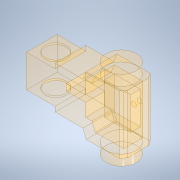
# Autodesk Inventor part: body_2
Saved by Autodesk Inventor 2020.2 (Build 242310000, 310)
## iProperties
Created: 2021-03-27
Part Number: body_2
Material: Generic
Document SubType Name: Modeling
Designer: DELL
Density: 1 g/cm^3
Appearance: Clear - Blue(1)
Author: DELL
Autodesk Inventor part; units mm, degrees
ref_plane "YZ Plane" through (0, 0, 0) normal (1, 0, 0) x (0, 1, 0)
ref_plane "XZ Plane" through (0, 0, 0) normal (0, 1, 0) x (-1, 0, 0)
sketch "Sketch1" plane through (0, 0, 0) normal (0, 0, 1) x (1, 0, 0)
  line L0 (-100, 0) -> (100, 0) construction
  line L1 (-100, 65) -> (-100, -65)
  circle A0 centre (-52.5, 57.5) radius 2.25
  line L2 (100, -70) -> (100, 70) construction
  line L3 (-92, 0) -> (-92, 57.5) construction
  line L4 (-92, 0) -> (-92, -57.5) construction
  circle A1 centre (-92.5, 57.5) radius 2.25
  circle A2 centre (-92.5, 57.5) radius 1.25
  circle A3 centre (-52.5, 57.5) radius 1.25
  line L5 (-100, 65) -> (-22.5777, 65)
  line L6 (-22.5777, 65) -> (-12.5777, 90)
  line L7 (-12.5777, 90) -> (100, 90)
  line L8 (100, 90) -> (100, 0)
  line L9 (100, -90) -> (100, 0)
  line L10 (-12.5777, -90) -> (100, -90)
  line L11 (-22.5777, -65) -> (-12.5777, -90)
  line L12 (-100, -65) -> (-22.5777, -65)
  line L13 (85, 75) -> (-2.4223, 75)
  line L14 (-2.4223, 75) -> (-12.4223, 50)
  line L15 (-12.4223, 50) -> (-92, 50)
  line L16 (-92, -50) -> (-12.4223, -50)
  line L17 (-12.4223, -50) -> (-2.4223, -75)
  line L18 (-2.4223, -75) -> (85, -75)
  line L19 (92.5, 82.5) -> (-7.5, 82.5) construction
  line L20 (-7.5, 82.5) -> (-17.5, 57.5) construction
  line L21 (-17.5, 57.5) -> (-92.5, 57.5) construction
  line L22 (-92.5, 57.5) -> (-92.5, -57.5) construction
  line L23 (-92.5, -57.5) -> (-17.5, -57.5) construction
  line L24 (-17.5, -57.5) -> (-7.5, -82.5) construction
  line L25 (-7.5, -82.5) -> (92.5, -82.5) construction
  line L26 (92.5, -82.5) -> (92.5, 0) construction
  line L27 (92.5, 0) -> (92.5, 82.5) construction
  line L28 (85, 75) -> (85, -75)
  line L29 (-100, 65) -> (-108, 65)
  line L30 (-108, 65) -> (-108, -65)
  line L31 (-108, -65) -> (-100, -65)
  line L32 (-100, -65) -> (-100, 65)
  line L33 (100, 0) -> (-108, 0)
  circle A4 centre (20, 82.5) radius 1.25
  circle A5 centre (20, 82.5) radius 2.25
  circle A6 centre (80, 82.5) radius 1.25
  circle A7 centre (80, 82.5) radius 2.25
  line L34 (50, 90) -> (50, 75) construction
  circle A8 centre (-12.5, 70) radius 1.25
  circle A9 centre (-12.5, 70) radius 2.25
  line L35 (-92, 50) -> (-92, -50)
  circle A10 centre (-96, 0) radius 2.25
  circle A11 centre (-96, 0) radius 1.25
  circle A12 centre (-104, 30) radius 2.25
  circle A13 centre (-104, 30) radius 1.25
  circle A14 centre (-104, -30) radius 2.25
  circle A15 centre (-104, -30) radius 1.25
  line L36 (-104, 65) -> (-104, -65) construction
  line L37 (-32, 50) -> (-32, 10)
  line L38 (-32, 10) -> (-92, 10)
  line L39 (77, 0) -> (77, -50)
  line L40 (77, -50) -> (-3, -50)
  line L41 (-3, -50) -> (-3, 0)
  line L42 (77, -40) -> (67, -40)
  line L43 (67, -40) -> (67, -50)
  line L44 (27, -50) -> (27, -40)
  line L45 (27, -40) -> (17, -40)
  line L46 (17, -40) -> (17, -50)
  circle A16 centre (57, 0) radius 7.5
  point P0 (0, 0)
  point P1 (0, 0)
  point P2 (77, 0)
  point P3 (-3, 0)
  dimension "d0" = 130
  dimension "d1" = 8
  dimension "d2" = 200
  dimension "d15" = 15
  dimension "d17" = 7.5
  dimension "d18" = 4.5
  dimension "d19" = 2.5
  dimension "d20" = 40
  dimension "d21" = 180
  dimension "d22" = 15
  dimension "d24" = 8
  dimension "d28" = 20
  dimension "d29" = 50
  dimension "d30" = 40
  dimension "d40" = 30
  dimension "d41" = 4
  dimension "d110" = 40
  dimension "d111" = 60
  dimension "d114" = 10
  dimension "d115" = 8
  dimension "d132" = 50
  dimension "d133" = 80
  dimension "d135" = 15
  dimension "d138" = 20
  dimension "d139" = 29
  dimension "d140" = 40
  dimension "d141" = 10
  constraints: 94 end point, 21 point on line, 17 centre point, 14 equal radius, 10 coincident, 8 perpendicular, 7 midpoint, 6 parallel, 6 symmetric about line, 4 vertical, 3 collinear, 3 equal length, 3 horizontal, 16 other
  measures "d0" distance of L29.start L12.start
  measures "d1" distance between parallel lines of L1 L3
  measures "d2" distance between parallel lines of L1 L2
  measures "d15" distance between parallel lines of L7 L13
  measures "d17" distance between parallel lines of L7 L19
  measures "d18" diameter of A1
  measures "d19" diameter of A2
  measures "d20" distance of A1.centre A3.centre
  measures "d21" distance between parallel lines of L10 L7
  measures "d22" distance between parallel lines of L9 L28
  measures "d24" distance between parallel lines of L1 L30
  measures "d28" distance from line of L8 A6.centre
  measures "d29" distance between parallel lines of L8 L34
  measures "d30" horizontal distance of A3.centre A8.centre
  measures "d40" distance from line of L33 A12.centre
  measures "d41" distance from line of L1 A10.centre
  measures "d110" distance of L37.start L37.end
  measures "d111" distance of L37.end L38.end
  measures "d114" distance of L42.end L43.end
  measures "d115" distance between parallel lines of L39 L28
  measures "d132" distance between parallel lines of L40 L0
  measures "d133" distance between parallel lines of L39 L41
  measures "d135" diameter of A16
  measures "d138" distance from line of L39 A16.centre
  measures "d139" distance between parallel lines of L37 L41
  measures "d140" distance between parallel lines of L44 L43
  measures "d141" horizontal distance of L6.start L6.end
sketch "Sketch6" plane through (0, 0, 0) normal (0, 0, 1) x (1, 0, 0)
  line L0 (0, -140.4945) -> (0, 142.9668) construction
  line L1 (59.9258, 0) -> (340.445, 0) construction
  line L2 (100, -70) -> (100, 70) construction
  line L3 (300, -100) -> (100, -70)
  line L4 (300, 100) -> (100, 70)
  dimension "d146" = 300
  dimension "d147" = 100
  constraints: 4 end point, 2 coincident, 1 symmetric about line
  measures "d146" distance from line of point (300, -100) L0
  measures "d147" distance from line of L1 point (300, -100)
ref_plane "Work Plane2" through (300, 100, 0) normal (-0.9889364, -0.1483405, 0) x (0.1483405, -0.9889364, 0)
sketch "Sketch7" plane through (300, 100, 0) normal (-0.9889364, -0.1483405, 0) x (0.1483405, -0.9889364, 0)
  circle A0 centre (0, 0) radius 2.5
  dimension "d150" = 5
  constraints: 1 centre point, 1 coincident
  measures "d150" diameter of A0
extrude "Extrusion1" add sketch "Sketch1" along normal mid plane 94 contours L5 L6 L7 L8 L33 L28 L13 L14 L15 L35 A10 L1 | L1 L33 L30 L29 | L33 A10 L35 L16 L17 L18 L28 L9 L10 L11 L12 L1 | L1 L31 L30 L33 | A10 L33 A11 | L33 A11 A10 | A11 L33 | L33 A11 | L35 L38 L37 L15 L14 L13 L28 L33 A16 | L33 L41 L40 L39 L28 L18 L17 L16 L35 | L33 A16 L39 L42 L43 L40 L44 L45 L46 L41 | L35 L15 L37 L38 | A16 L33 | L33 A16 | L46 L45 L44 L40 | L39 L40 L43 L42 | A0 | A1 | A2 | A3 | A4 | A5 | A6 | A7 | A8 | A9 | A12 | A13 | A14 | A15
extrude "Extrusion2" cut sketch "Sketch1" along normal mid plane 59 contours L35 L38 L37 L15 L14 L13 L28 L33 A16 | L33 L41 L40 L39 L28 L18 L17 L16 L35 | L33 A16 L39 L42 L43 L40 L44 L45 L46 L41 | L35 L15 L37 L38 | A16 L33 | L33 A16 | L46 L45 L44 L40 | L39 L40 L43 L42
sketch "Sketch2" plane through (-108, -65, 47) normal (-1, 0, 0) x (0, 0, 1)
  line L0 (0, -25) -> (0, 155) projected
  line L1 (-94, 15) -> (0, 15)
  line L2 (0, 15) -> (0, 115)
  line L3 (0, 115) -> (-94, 115)
  line L4 (-94, 115) -> (-94, 15)
  line L5 (-94, 15) -> (0, 115) construction
  line L6 (0, 15) -> (-94, 115) construction
  line L7 (-94, 42) -> (0, 42)
  line L8 (0, 42) -> (0, 88)
  line L9 (0, 88) -> (-94, 88)
  line L10 (-94, 88) -> (-94, 42)
  line L11 (-94, 42) -> (0, 88) construction
  line L12 (0, 42) -> (-94, 88) construction
  point P0 (-47, 65)
  dimension "d52" = 100
  dimension "d55" = 46
  constraints: 24 end point, 4 midpoint, 4 parallel, 2 horizontal, 2 perpendicular, 2 point on line
  measures "d52" distance between parallel lines of L1 L3
  measures "d55" distance between parallel lines of L7 L9
extrude "Extrusion3" add sketch "Sketch2" along normal blind 88
extrude "Extrusion4" [suppressed]
sketch "Sketch3" plane through (0, 0, 0) normal (0, 1, 0) x (-1, 0, 0)
  circle A0 centre (153, 0) radius 32.5
  line L0 (108, -47) -> (108, 47) projected
  line L1 (108, -47) -> (108, 47) projected
  line L2 (108, -47) -> (108, 47) construction
  line L3 (108, 0) -> (245.8238, 0) construction
  circle A1 centre (153, 0) radius 40
  line L4 (183.942, 9.942) -> (196, 22)
  line L5 (196, 22) -> (196, -22)
  line L6 (196, -22) -> (183.942, -9.942)
  line L7 (196, 47) -> (196, -47) projected
  line L8 (204, 47) -> (224, 20)
  line L9 (224, 20) -> (224, 47)
  line L10 (224, 47) -> (204, 47)
  line L11 (196, -47) -> (224, -47)
  line L12 (204, -47) -> (224, -20)
  line L13 (224, -20) -> (224, -47)
  line L14 (-100, 47) -> (12.5777, 47) projected
  line L15 (-100, 47) -> (-100, 32)
  line L16 (-100, 32) -> (-90, 47)
  line L17 (-100, -47) -> (12.5777, -47)
  line L18 (-100, -47) -> (-100, -32)
  line L19 (-100, -32) -> (-90, -47)
  circle A2 centre (-48, 0) radius 46
  line L20 (-100, 47) -> (-100, -47) projected
  circle A3 centre (-48, 0) radius 32.5
  line L21 (-4.8723, -16) -> (13.1277, -16)
  line L22 (13.1277, -16) -> (13.1277, 16)
  line L23 (13.1277, 16) -> (-4.8723, 16)
  point P0 (0, 0)
  point P1 (189.7631, 15.7631)
  point P2 (189.7631, -15.7631)
  dimension "d58" = 45
  dimension "d59" = 65
  dimension "d62" = 80
  dimension "d64" = 44
  dimension "d69" = 20
  dimension "d70" = 27
  dimension "d80" = 15
  dimension "d81" = 10
  dimension "d87" = 52
  dimension "d88" = 92
  dimension "d116" = 65
  dimension "d121" = 32
  dimension "d122" = 18
  dimension "d134" = 8
  dimension "d143" = 48
  constraints: 36 end point, 7 symmetric about line, 5 point on line, 4 centre point, 4 point on circle, 3 perpendicular, 3 vertical, 2 coincident, 2 horizontal, 1 collinear, 1 horizontal alignment, 1 midpoint, 2 other
  measures "d58" distance from line of L0 A0.centre
  measures "d59" diameter of A0
  measures "d62" diameter of A1
  measures "d64" distance of L4.end L5.end
  measures "d69" horizontal distance of L8.start L8.end
  measures "d70" vertical distance of L8.start L8.end
  measures "d80" distance of L14.start L15.end
  measures "d81" horizontal distance of L15.end L16.end
  measures "d87" distance from line of L20 A2.centre
  measures "d88" diameter of A2
  measures "d116" diameter of A3
  measures "d121" distance of L21.end L22.end
  measures "d122" distance of L22.end L23.end
  measures "d134" distance of L7.start L8.start
  measures "d143" distance of point (0, 0) A2.centre
extrude "Extrusion15" cut sketch "Sketch3" along normal through all both and the other way through all contours L10 L9 L8 | L12 L13 L11 | L14 L16 L15 | L18 L19 L17
extrude "Extrusion16" add sketch "Sketch1" along normal through all both and the other way through all contours L35 L15 L37 L38
extrude "Extrusion14" add sketch "Sketch3" against normal blind 32 from surface at -90 contours A2 | A3
extrude "Extrusion17" [suppressed]
extrude "Extrusion18" cut sketch "Sketch3" along normal blind 5 from surface at -50 contours A0
extrude "Extrusion21" cut sketch "Sketch1" along normal up to surface (17.5 mm away) from surface at -47 contours A16 L33 | L33 A16
extrude "Extrusion22" add sketch "Sketch1" along normal blind 30 from surface at -29.5 contours L33 A16 L39 L42 L43 L40 L44 L45 L46 L41 | L33 A16 | L46 L45 L44 L40 | L39 L40 L43 L42 picked at (58.4928, -2.6557)
extrude "Extrusion24" [suppressed]
mirror "Mirror2" about plane through (0, 0, 0) normal (0, 1, 0) of "Extrusion14", "Extrusion16", "Extrusion18", "Extrusion22"
equation "\"d17\" = 0.5 * d15"
equation "\"d21\" = d47"
equation "\"d45\" = 124"
equation "\"d46\" = 12"
equation "\"d47\" = 180"
body "Solid1"
